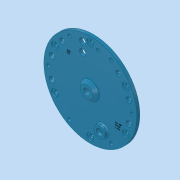
# Autodesk Inventor part: aftSpoolSectionSealingWall
Saved by Autodesk Inventor 2017 (Build 210142000, 142)
## iProperties
Created: 2016-11-06
Part Number: aftSpoolSectionSealingWall
Material: ABS Plastic
Document SubType Name: Modeling
Designer: techn
Density: 1.06 g/cm^3
Appearance: Sky Blue Dark
Mass: 23.728 g
Surface Area: 158.495 cm^2
Volume: 22.3849 cm^3
Author: techn
Autodesk Inventor part; units mm, degrees
ref_plane "YZ Plane" through (0, 0, 0) normal (1, 0, 0) x (0, 1, 0)
ref_plane "XZ Plane" through (0, 0, 0) normal (0, 1, 0) x (-1, 0, 0)
ref_plane "XY Plane" through (0, 0, 0) normal (0, 0, 1) x (1, 0, 0)
sketch "Sketch1" plane through (0, 0, 0) normal (0, 0, 1) x (1, 0, 0)
  circle A0 centre (0, 0) radius 47.625
  dimension "d0" = 95.25
  constraints: 1 centre point, 1 coincident
  measures "d0" diameter of A0
extrude "Extrusion1" add sketch "Sketch1" along normal blind 3.175
sketch "Sketch4" plane through (0, 0, 3.175) normal (0, 0, 1) x (1, 0, 0)
  circle A0 centre (12.446, -29.7561) radius 3.3655
  point P0 (0, 0)
  dimension "d16" = 6.731
  dimension "d17" = 12.446
  dimension "d18" = 29.7561
  constraints: 1 centre point
  measures "d16" diameter of A0
  measures "d17" horizontal distance of A0.centre point (0, 0)
  measures "d18" vertical distance of A0.centre point (0, 0)
extrude "Extrusion4" cut sketch "Sketch4" against normal blind 3.175
sketch "Sketch6" plane through (0, 0, 3.175) normal (0, 0, 1) x (1, 0, 0)
  circle A0 centre (0, 0) radius 3.3655
  circle A1 centre (0, 0) radius 9.525
  circle A2 centre (0, 0) radius 47.625 projected
  circle A3 centre (12.446, -29.7561) radius 3.3655 projected
  line L0 (0, 0) -> (12.446, -29.7561) construction
  dimension "d32" = 6.731
  dimension "d33" = 19.05
  dimension "d191" = 32.2541
  constraints: 3 coincident, 2 centre point, 2 end point
  measures "d32" diameter of A0
  measures "d33" diameter of A1
  measures "d191" distance of L0.start L0.end
extrude "Extrusion7" add sketch "Sketch6" along normal blind 3.81 contours A1
sketch "Sketch7" plane through (0, 0, 3.175) normal (0, 0, 1) x (1, 0, 0)
  line L0 (0, 0) -> (21.4313, 37.12)
  line L1 (0, 0) -> (42.8625, 0) construction
  circle A0 centre (21.4313, 37.12) radius 1.8415
  circle A1 centre (-21.4312, 37.12) radius 1.8415
  circle A2 centre (-42.8625, 0) radius 1.8415
  circle A3 centre (-21.4313, -37.12) radius 1.8415
  circle A4 centre (21.4312, -37.12) radius 1.8415
  circle A5 centre (42.8625, 0) radius 1.8415
  dimension "d39" = 42.8625
  dimension "d40" = 60
  dimension "d41" = 3.683
  dimension "d44" = 360
  constraints: 6 centre point, 4 end point, 1 coincident, 1 equal length, 1 horizontal, 13 other
  measures "d39" distance of L0.start L0.end
  measures "d40" angle of L1 L0
  measures "d41" diameter of A0
extrude "Extrusion10" cut sketch "Sketch7" against normal through all
sketch "Sketch9" plane through (0, 0, 3.175) normal (0, 0, 1) x (1, 0, 0)
  circle A0 centre (0, 0) radius 3.3655 projected
  line L0 (0, 0) -> (0, 41.91)
  circle A1 centre (0, 41.91) radius 1.8415
  circle A2 centre (-36.2951, 20.955) radius 1.8415
  circle A3 centre (-36.2951, -20.955) radius 1.8415
  circle A4 centre (0, -41.91) radius 1.8415
  circle A5 centre (36.2951, -20.955) radius 1.8415
  circle A6 centre (36.2951, 20.955) radius 1.8415
  dimension "d61" = 41.91
  dimension "d62" = 3.683
  dimension "d65" = 360
  constraints: 6 centre point, 2 end point, 1 coincident, 1 vertical, 13 other
  measures "d61" distance of L0.start L0.end
  measures "d62" diameter of A1
extrude "Extrusion12" cut sketch "Sketch9" against normal blind 25.4 contours A1 | A2 | A3 | A4 | A5 | A6
sketch "Sketch17" plane through (0, 0, 3.175) normal (0, 0, 1) x (1, 0, 0)
  line L0 (0, 0) -> (39.3779, 10.5513)
  line L1 (0, 0) -> (40.767, 0) construction
  circle A0 centre (39.3779, 10.5513) radius 2.794
  line L2 (0, 0) -> (0, 17.3134)
  circle A1 centre (39.3779, -10.5513) radius 2.794
  circle A2 centre (-39.3779, 10.5513) radius 2.794
  circle A3 centre (-39.3779, -10.5513) radius 2.794
  line L3 (0, 0) -> (28.8266, 28.8266)
  line L4 (0, 0) -> (40.767, 0) construction
  circle A4 centre (28.8266, 28.8266) radius 2.794
  circle A5 centre (-28.8266, 28.8266) radius 2.794
  dimension "d144" = 40.767
  dimension "d145" = 15
  dimension "d146" = 5.588
  dimension "d149" = 40.767
  dimension "d150" = 45
  dimension "d151" = 5.588
  constraints: 10 end point, 6 centre point, 4 symmetric about line, 2 coincident, 2 equal length, 2 horizontal, 1 vertical, 4 other
  measures "d144" distance of L0.start L0.end
  measures "d145" angle of L1 L0
  measures "d146" diameter of A0
  measures "d149" distance of L0.start L3.end
  measures "d150" angle of L4 L3
  measures "d151" diameter of A4
extrude "Extrusion22" cut sketch "Sketch17" against normal blind 25.4 contours A0 | A1 | A2 | A3
extrude "Extrusion23" cut sketch "Sketch17" against normal blind 25.4 contours A4 | A5
sketch "Sketch22" plane through (0, 0, 3.175) normal (0, 0, 1) x (1, 0, 0)
  circle A0 centre (-7.9375, 29.1338) radius 3.3655
  point P0 (0, 0)
  dimension "d166" = 6.731
  dimension "d167" = 7.9375
  dimension "d168" = 29.1338
  constraints: 1 centre point
  measures "d166" diameter of A0
  measures "d167" horizontal distance of point (0, 0) A0.centre
  measures "d168" vertical distance of point (0, 0) A0.centre
extrude "Extrusion26" cut sketch "Sketch22" against normal through all
sketch "Sketch23" plane through (0, 0, 3.175) normal (0, 0, 1) x (1, 0, 0)
  circle A0 centre (0, 0) radius 3.3655 projected
extrude "Extrusion27" cut sketch "Sketch23" against normal blind 1.5875
chamfer "Chamfer6" distance 3.175 angle 45 1 edges at (-9.525, 0, 6.985)
sketch "Sketch24" plane through (0, 0, 3.175) normal (0, 0, 1) x (1, 0, 0)
  circle A0 centre (12.446, -29.7561) radius 3.3655 projected
  circle A1 centre (12.446, -29.7561) radius 5.715
  point P0 (0, 0)
  dimension "d176" = 11.43
  constraints: 1 centre point, 1 coincident
  measures "d176" diameter of A1
extrude "Extrusion28" add sketch "Sketch24" along normal blind 3.175
sketch "Sketch25" plane through (0, 0, 0) normal (0, 0, -1) x (-1, 0, 0)
  circle A0 centre (-12.446, -29.7561) radius 3.3655 projected
  circle A1 centre (-12.446, -29.7561) radius 1.905
  point P0 (0, 0)
  dimension "d179" = 3.81
  constraints: 1 centre point, 1 coincident
  measures "d179" diameter of A1
extrude "Extrusion29" add sketch "Sketch25" against normal blind 3.175
fillet "Fillet3" radius 1.27 1 edges at (6.731, -29.7561, 3.175)
sketch "Sketch26" plane through (0, 0, 3.175) normal (0, 0, 1) x (1, 0, 0)
  circle A0 centre (-7.9375, 38.862) radius 3.3655
  circle A1 centre (7.9375, 38.862) radius 1.905
  line L0 (7.9375, 38.862) -> (-7.9375, 38.862) construction
  circle A2 centre (-7.9375, 29.1338) radius 3.3655 construction
  line L1 (-7.9375, 29.1338) -> (-7.9375, 38.862) construction
  point P0 (0, 0)
  point P1 (0, 38.862)
  dimension "d183" = 6.731
  dimension "d184" = 3.81
  dimension "d185" = 38.862
  dimension "d186" = 15.875
  dimension "d189" = 9.7282
  constraints: 4 end point, 2 centre point, 1 horizontal, 1 midpoint, 1 vertical alignment
  measures "d183" diameter of A0
  measures "d184" diameter of A1
  measures "d185" vertical distance of point (0, 0) L0.start
  measures "d186" distance of L0.end L0.start
  measures "d189" distance of L1.start L0.end
extrude "Extrusion30" cut sketch "Sketch26" against normal through all
sketch "Sketch27" plane through (0, 0, 3.175) normal (0, 0, 1) x (1, 0, 0)
  line L0 (-24.0461, 24.2224) -> (-19.7824, 24.2224) construction
  line L1 (-19.7824, 24.2224) -> (-19.7824, 20.2457) construction
  line L2 (-19.7824, 20.2457) -> (-24.0461, 20.2457) construction
  line L3 (-24.0461, 20.2457) -> (-24.0461, 24.2224) construction
  line L4 (25.5336, -15.2981) -> (30.1056, -15.2981) construction
  line L5 (30.1056, -15.2981) -> (30.1056, -17.0126) construction
  line L6 (30.1056, -17.0126) -> (25.5336, -17.0126) construction
  line L7 (25.5336, -17.0126) -> (25.5336, -15.2981) construction
  constraints: 4 other
sketch "Sketch29" plane through (0, 0, 3.175) normal (0, 0, 1) x (1, 0, 0)
  circle A0 centre (0, 41.91) radius 1.8415 projected
  circle A1 centre (0, 41.91) radius 3.683
  point P0 (0, 0)
  dimension "d192" = 7.366
  constraints: 1 centre point, 1 coincident
  measures "d192" diameter of A1
extrude "Extrusion31" cut sketch "Sketch29" against normal blind 1.27
pattern_circular "Circular Pattern1" count 6 over 360 about axis through (0, 0, 0) along (0, 0, 1) of "Extrusion31"
sketch "Sketch21" plane through (0, 0, 0) normal (0, 0, -1) x (-1, 0, 0)
  circle A0 centre (0, 0) radius 47.625
  circle A1 centre (0, 0) radius 9.525 projected
  circle A2 centre (0, 0) radius 47.1805
  dimension "d162" = 95.25
  dimension "d163" = 94.361
  constraints: 2 centre point, 2 coincident
  measures "d162" diameter of A0
  measures "d163" diameter of A2
extrude "PRINT_FEATURE_1" [suppressed]
body "Solid1"
